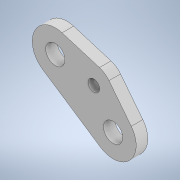
# Autodesk Inventor part: wspornik_amortyzatora
Saved by Autodesk Inventor 2020.3 (Build 243373000, 373)
## iProperties
Created: 2021-11-02
Part Number: wspornik_amortyzatora
Material: Ogólny
Document SubType Name: Modeling
Designer: patry
Density: 1 g/cm^3
Appearance: Domyślna
Author: patry
Autodesk Inventor part; units mm, degrees
ref_plane "YZ Plane" through (0, 0, 0) normal (1, 0, 0) x (0, 1, 0)
ref_plane "XZ Plane" through (0, 0, 0) normal (0, 1, 0) x (-1, 0, 0)
ref_plane "XY Plane" through (0, 0, 0) normal (0, 0, 1) x (1, 0, 0)
sketch "Szkic1" plane through (0, 0, 0) normal (0, 0, 1) x (1, 0, 0)
  circle A0 centre (0.3365, 7.2308) radius 5
  circle A1 centre (-9.6635, 9.2308) radius 6
  circle A2 centre (5.3365, -0.7692) radius 6
  line L0 (-7.9155, 14.9705) -> (1.7932, 12.0139)
  line L1 (4.2717, 10.3153) -> (10.0588, 2.9322)
  line L2 (-12.9917, 4.2385) -> (2.0083, -5.7615)
  point P0 (0, 0)
  dimension "d0" = 15
  dimension "d1" = 10
  dimension "d2" = 8
  dimension "d3" = 5
  dimension "d4" = 10
  dimension "d5" = 12
  dimension "d6" = 12
  constraints: 6 end point, 6 point on circle, 6 tangent, 3 centre point, 3 coincident
  measures "d0" horizontal distance of point (5.337, -0.769) point (-9.663, 9.231)
  measures "d1" vertical distance of point (5.337, -0.769) point (-9.663, 9.231)
  measures "d2" vertical distance of point (5.337, -0.769) point (0.337, 7.231)
  measures "d3" horizontal distance of point (5.337, -0.769) point (0.337, 7.231)
  measures "d4" diameter of A0
  measures "d5" diameter of A1
  measures "d6" diameter of A2
extrude "Wyciągnięcie proste1" add sketch "Szkic1" along normal blind 3
hole "Otwór1" at (5.3365, -0.7692, 0) at (-9.6635, 9.2308, 0) direction (0, 0, 1) diameter 5 end through all
hole "Otwór2" at (0.3365, 7.2308, 0) direction (0, 0, 1) diameter 3 end through all
